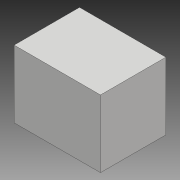
# Autodesk Inventor part: case
Saved by Autodesk Inventor 2017 (Build 210142000, 142)
## iProperties
Created: 2022-04-09
Part Number: case
Material: Generic
Document SubType Name: Modeling
Designer: jocke
Density: 1 g/cm^3
Appearance: Default
Author: jocke
Autodesk Inventor part; units mm, degrees
ref_plane "YZ Plane" through (0, 0, 0) normal (1, 0, 0) x (0, 1, 0)
ref_plane "XZ Plane" through (0, 0, 0) normal (0, 1, 0) x (-1, 0, 0)
ref_plane "XY Plane" through (0, 0, 0) normal (0, 0, 1) x (1, 0, 0)
sketch "Sketch1" plane through (0, 0, 0) normal (0, 1, 0) x (-1, 0, 0)
  line L0 (0, 0) -> (-136, 0)
  line L1 (-136, 0) -> (-136, 106)
  line L2 (-136, 106) -> (0, 106)
  line L3 (0, 106) -> (0, 0)
  dimension "d0" = 106
  dimension "d1" = 136
  constraints: 8 end point, 2 parallel, 1 horizontal, 1 perpendicular
  measures "d0" distance of L0.end L1.end
  measures "d1" distance of L1.end L2.end
extrude "Extrusion1" add sketch "Sketch1" along normal blind 3
sketch "Sketch2" plane through (0, 3, 0) normal (0, 1, 0) x (1, 0, 0)
  line L0 (3, -3) -> (133, -3)
  line L1 (133, -3) -> (133, -103)
  line L2 (133, -103) -> (3, -103)
  line L3 (3, -103) -> (3, -3)
  line L4 (0, 0) -> (0, -106) projected
  line L5 (136, 0) -> (0, 0) projected
  line L6 (0, -106) -> (136, -106) projected
  line L7 (0, 0) -> (136, 0)
  line L8 (136, 0) -> (136, -106)
  line L9 (136, -106) -> (0, -106)
  line L10 (0, -106) -> (0, 0)
  dimension "d4" = 130
  dimension "d5" = 100
  dimension "d6" = 3
  dimension "d7" = 3
  constraints: 16 end point, 4 parallel, 2 horizontal, 2 perpendicular
  measures "d4" distance of L0.start L0.end
  measures "d5" distance of L0.end L1.end
  measures "d6" distance between parallel lines of L4 L3
  measures "d7" distance between parallel lines of L5 L0
extrude "Extrusion2" add sketch "Sketch2" along normal blind 100
body "Solid1"
